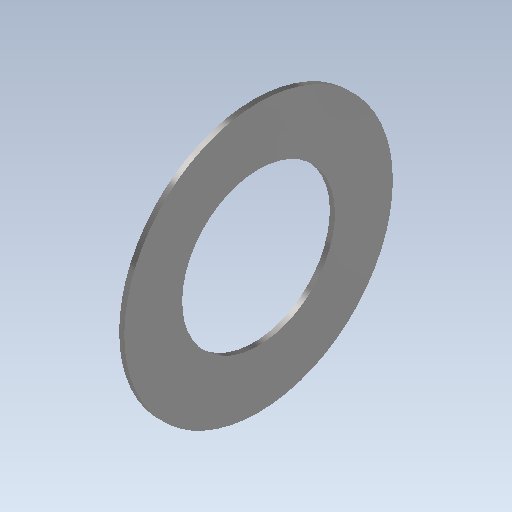
# Autodesk Inventor part: F694ZZ Shield2
Saved by Autodesk Inventor 2020 (Build 240168000, 168)
## iProperties
Created: 2018-10-12
Part Number: F694ZZ Shield2
Material: ステンレス鋼 440C
Catalog Web Link: www.cadenas.de
Description: shielded_type_zz_zzs_S2-
Vendor: NSK_RB
Document SubType Name: Modeling
Designer: psadmin
Manufacturer: NSK_RB
Mass: 0.0748994 g
Surface Area: 1.12238 cm^2
Volume: 0.00966444 cm^3
Density: 7.75 g/cm^3
Appearance: 半つや出し
Category: PARTsolutions
Company: NSK_RB
PSOL_IDENT_0: {$CADENAS_DATA\23d-libs\nsk_rb\roller_bearings\deep_groove_bb\exstra_small_miniatur_bb\metric_design
PSOL_IDENT_1: _with_flange\shielded_type_zz_zzs_s2_1.prj},186 {VTYP=3D},{NB=F694ZZ Shield2},{LINA=F694ZZ Shield2},
PSOL_IDENT_2: {NN=shielded_type_zz_zzs_S2},{DATE=18.07.2018 08:51:06},{GEOMDATE=04.01.2008 00:00:00},{VERSION=},{L
PSOL_IDENT_3: INEID=250},{WBVAR=},{WBNUMERIC=}  {NB=F694ZZ Shield2},{LINA=F694ZZ Shield2},{KT=DUMMY},{IDNR=},{STAN=
PSOL_IDENT_4: },{ORDER=F694ZZ},{SD=4.0},{X=4.0},{D=11},{DD=11},{DD1=0.0},{D2=12.5},{DD2=12.5},{B=0.0},{B1=4.0},{CC
PSOL_IDENT_5: 1=0.0},{C2=1.0},{CC2=1.0},{R=0.00},{R1=0.15},{DI1=6.15},{DI2=5.60},{SDE1=8.95},{SDE2=9.85},{CR1=960}
PSOL_IDENT_6: ,{COR1=345},{CR2=98},{COR2=35.0},{LG=48000},{LO=56000},{DA=0.0},{DB=5.6},{RA=0.00},{RB=0.15},{MASS=1
PSOL_IDENT_7: .96},{SC=1}
NN: shielded_type_zz_zzs_S2
NB: F694ZZ Shield2
NBSYN: $ORDER. Shield2
LINA: F694ZZ Shield2
ORDER: F694ZZ
SD: 4
X: 4
D: 11
DD: 11
DD1: 0
D2: 12.5
DD2: 12.5
B: 0
B1: 4
CC1: 0
C2: 1
CC2: 1
R: 0
R1: 0.15
DI1: 6.15
DI2: 5.6
SDE1: 8.95
SDE2: 9.85
CR1: 960
COR1: 345
CR2: 98
COR2: 35
LG: 48000
LO: 56000
DA: 0
DB: 5.6
RA: 0
RB: 0.15
MASS: 1.96
SC: 1
SUPPLIER: NSK_RB
ARTICLENO: F694ZZ Shield2
BOMINFO: F694ZZ Shield2
CREATOR: CADENAS GmbH
Title: F694ZZ Shield2
Author: Cadenas PARTsolutions
Autodesk Inventor part; units mm, degrees
sketch "Sketch_1" plane through (0, 0, 0) normal (0, 0, 1) x (1, 0, 0)
  line L0 (3.9374, 0) -> (3.75, 0)
  line L1 (3.75, 2.8) -> (3.9374, 2.8)
  line L2 (3.9374, 2.8) -> (3.9374, 4.925)
  line L3 (3.9374, 4.925) -> (3.75, 4.925)
  line L4 (3.75, 4.925) -> (3.75, 2.8)
  constraints: 10 end point
revolve "Revolution1" add sketch "Sketch_1" angle 360 about axis through (3.9374, 0, 0) along (1, 0, 0)
ref_plane "ip_st_1_XY" through (3.75, 0, 0) normal (1, 0, 0) x (0, 0, -1)
ref_plane "ip_st_1_YZ" through (3.75, 0, 0) normal (0, 0, -1) x (0, 1, 0)
ref_plane "ip_st_1_ZX" through (3.75, 0, 0) normal (0, 1, 0) x (1, 0, 0)
body "Solid1"
